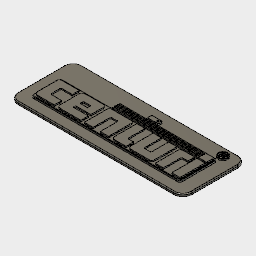
Centuri (Autodesk Fusion 360 design; units mm, degrees)
Autodesk Fusion 360 part; units mm, degrees
sketch "Sketch1" plane through (0, 0, 0) normal (0, 1, 0) x (1, 0, 0)
  spline S0 degree 3 poles (174.1224, -9.0926) (174.1224, -4.1474) (170.1072, -0.1324) (165.162, -0.1324) knots 0 0 0 0 1 1 1 1
  line L0 (165.162, -0.1324) -> (9.0926, -0.1324)
  spline S1 degree 3 poles (9.0926, -0.1324) (4.1474, -0.1324) (0.1323, -4.1474) (0.1323, -9.0926) knots 0 0 0 0 1 1 1 1
  line L1 (0.1323, -9.0926) -> (0.1323, -55.1748)
  spline S2 degree 3 poles (0.1323, -55.1748) (0.1323, -60.12) (4.1474, -64.135) (9.0926, -64.135) knots 0 0 0 0 1 1 1 1
  line L2 (9.0926, -64.135) -> (165.162, -64.135)
  spline S3 degree 3 poles (165.162, -64.135) (170.1072, -64.135) (174.1224, -60.12) (174.1224, -55.1748) knots 0 0 0 0 1 1 1 1
  line L3 (174.1224, -55.1748) -> (174.1224, -9.0926)
extrude "Extrude1" add sketch "Sketch1" along normal blind 2.5
sketch "Sketch2" plane through (0, 2.5, 0) normal (0, 1, 0) x (-1, 0, 0)
  line L0 (-174.1224, 55.1748) -> (-174.1224, 9.0926)
  spline S0 degree 3 poles (-174.1224, 9.0926) (-174.1224, 4.1474) (-170.1072, 0.1324) (-165.162, 0.1324) knots 0 0 0 0 1 1 1 1
  line L1 (-165.162, 0.1324) -> (-9.0926, 0.1324)
  spline S1 degree 3 poles (-9.0926, 0.1324) (-4.1474, 0.1324) (-0.1323, 4.1474) (-0.1323, 9.0926) knots 0 0 0 0 1 1 1 1
  line L2 (-0.1323, 9.0926) -> (-0.1323, 55.1748)
  spline S2 degree 3 poles (-0.1323, 55.1748) (-0.1323, 60.12) (-4.1474, 64.135) (-9.0926, 64.135) knots 0 0 0 0 1 1 1 1
  line L3 (-9.0926, 64.135) -> (-165.162, 64.135)
  spline S3 degree 3 poles (-165.162, 64.135) (-170.1072, 64.135) (-174.1224, 60.12) (-174.1224, 55.1748) knots 0 0 0 0 1 1 1 1
  spline S4 degree 2 poles (-15.1624, 24.5465) (-23.495, 24.5465) (-62.1665, 24.5613) knots 0 0 0 1 1 1
  spline S5 degree 2 poles (-62.1665, 24.5613) (-62.5856, 24.583) (-62.9216, 24.4382) knots 0 0 0 1 1 1
  spline S6 degree 3 poles (-62.9216, 24.4382) (-62.998, 24.4054) (-63.1803, 24.2591) (-63.2581, 24.0509) knots 0 0 0 0 1 1 1 1
  spline S7 degree 2 poles (-63.2581, 24.0509) (-63.3521, 23.7995) (-63.3351, 23.482) knots 0 0 0 1 1 1
  spline S8 degree 2 poles (-63.3351, 23.482) (-63.338, 19.0394) (-63.3351, 17.8062) knots 0 0 0 1 1 1
  spline S9 degree 3 poles (-63.3351, 17.8062) (-63.3335, 17.1487) (-63.7825, 16.1729) (-64.44, 16.1721) knots 0 0 0 0 1 1 1 1
  spline S10 degree 3 poles (-64.44, 16.1721) (-68.6437, 16.1658) (-83.8279, 16.1713) (-88.5401, 16.1711) knots 0 0 0 0 1 1 1 1
  spline S11 degree 3 poles (-88.5401, 16.1711) (-89.2008, 16.1708) (-89.5479, 16.224) (-89.5627, 15.5723) knots 0 0 0 0 1 1 1 1
  spline S12 degree 2 poles (-89.5627, 15.5723) (-89.5961, 14.1198) (-89.5627, 11.2842) knots 0 0 0 1 1 1
  spline S13 degree 3 poles (-89.5627, 11.2842) (-89.5627, 10.7958) (-89.9593, 10.3992) (-90.4478, 10.3992) knots 0 0 0 0 1 1 1 1
  line L4 (-90.4478, 10.3992) -> (-99.1457, 10.3992)
  spline S14 degree 3 poles (-99.1457, 10.3992) (-99.6341, 10.3992) (-100.0307, 10.7958) (-100.0307, 11.2842) knots 0 0 0 0 1 1 1 1
  spline S15 degree 2 poles (-100.0307, 11.2842) (-100.0021, 14.3261) (-100.0209, 15.5535) knots 0 0 0 1 1 1
  spline S16 degree 3 poles (-100.0209, 15.5535) (-100.0315, 16.242) (-100.4882, 16.1708) (-101.101, 16.1716) knots 0 0 0 0 1 1 1 1
  spline S17 degree 3 poles (-101.101, 16.1716) (-110.8882, 16.1846) (-148.8429, 16.1753) (-158.7502, 16.1721) knots 0 0 0 0 1 1 1 1
  spline S18 degree 3 poles (-158.7502, 16.1721) (-159.6421, 16.1716) (-160.4602, 17.3384) (-160.4594, 18.2301) knots 0 0 0 0 1 1 1 1
  spline S19 degree 3 poles (-160.4594, 18.2301) (-160.4576, 20.1639) (-160.4679, 26.0257) (-160.4679, 27.4458) knots 0 0 0 0 1 1 1 1
  spline S20 degree 2 poles (-160.4679, 27.4458) (-160.4674, 46.2841) (-160.4679, 50.641) knots 0 0 0 1 1 1
  spline S21 degree 3 poles (-160.4679, 50.641) (-160.4682, 53.0103) (-159.9139, 53.5406) (-157.5686, 53.5406) knots 0 0 0 0 1 1 1 1
  spline S22 degree 3 poles (-157.5686, 53.5406) (-133.3068, 53.5403) (-39.3625, 53.5421) (-15.1624, 53.5406) knots 0 0 0 0 1 1 1 1
  spline S23 degree 3 poles (-15.1624, 53.5406) (-12.6611, 53.5403) (-11.9475, 53.0579) (-11.9488, 50.641) knots 0 0 0 0 1 1 1 1
  spline S24 degree 3 poles (-11.9488, 50.641) (-11.9515, 46.2857) (-11.9491, 31.8307) (-11.9488, 27.4458) knots 0 0 0 0 1 1 1 1
  spline S25 degree 3 poles (-11.9488, 27.4458) (-11.9488, 25.0253) (-12.6291, 24.5465) (-15.1624, 24.5465) knots 0 0 0 0 1 1 1 1
extrude "Extrude2" add sketch "Sketch2" along normal blind 2 contours S4 S5 S6 S7 S8 S9 S10 S11 S12 S13 L4 S14 S15 S16 S17 S18 S19 S20 S21 S22 S23 S24 S25
sketch "Sketch3" plane through (0, 4.5, 0) normal (0, 1, 0) x (-1, 0, 0)
  spline S0 degree 3 poles (-11.9488, 27.4458) (-11.9491, 31.8307) (-11.9515, 46.2857) (-11.9488, 50.641) knots -1 -1 -1 -1 0 0 0 0
  spline S1 degree 3 poles (-11.9488, 50.641) (-11.9475, 53.0579) (-12.6611, 53.5403) (-15.1624, 53.5406) knots -1 -1 -1 -1 0 0 0 0
  spline S2 degree 3 poles (-15.1624, 53.5406) (-39.3625, 53.5421) (-133.3068, 53.5403) (-157.5686, 53.5406) knots -1 -1 -1 -1 0 0 0 0
  spline S3 degree 3 poles (-157.5686, 53.5406) (-159.9139, 53.5406) (-160.4682, 53.0103) (-160.4679, 50.641) knots -1 -1 -1 -1 0 0 0 0
  spline S4 degree 2 poles (-160.4679, 50.641) (-160.4674, 46.2841) (-160.4679, 27.4458) knots -1 -1 -1 0 0 0
  spline S5 degree 3 poles (-160.4679, 27.4458) (-160.4679, 26.0257) (-160.4576, 20.1639) (-160.4594, 18.2301) knots -1 -1 -1 -1 0 0 0 0
  spline S6 degree 3 poles (-160.4594, 18.2301) (-160.4602, 17.3384) (-159.6421, 16.1716) (-158.7502, 16.1721) knots -1 -1 -1 -1 0 0 0 0
  spline S7 degree 3 poles (-158.7502, 16.1721) (-148.8429, 16.1753) (-110.8882, 16.1846) (-101.101, 16.1716) knots -1 -1 -1 -1 0 0 0 0
  spline S8 degree 3 poles (-101.101, 16.1716) (-100.4882, 16.1708) (-100.0315, 16.242) (-100.0209, 15.5535) knots -1 -1 -1 -1 0 0 0 0
  spline S9 degree 2 poles (-100.0209, 15.5535) (-100.0021, 14.3261) (-100.0307, 11.2842) knots -1 -1 -1 0 0 0
  spline S10 degree 3 poles (-100.0307, 11.2842) (-100.0307, 10.7958) (-99.6341, 10.3992) (-99.1457, 10.3992) knots -1 -1 -1 -1 0 0 0 0
  line L0 (-99.1457, 10.3992) -> (-90.4478, 10.3992)
  spline S11 degree 3 poles (-90.4478, 10.3992) (-89.9593, 10.3992) (-89.5627, 10.7958) (-89.5627, 11.2842) knots -1 -1 -1 -1 0 0 0 0
  spline S12 degree 2 poles (-89.5627, 11.2842) (-89.5961, 14.1198) (-89.5627, 15.5723) knots -1 -1 -1 0 0 0
  spline S13 degree 3 poles (-89.5627, 15.5723) (-89.5479, 16.224) (-89.2008, 16.1708) (-88.5401, 16.1711) knots -1 -1 -1 -1 0 0 0 0
  spline S14 degree 3 poles (-88.5401, 16.1711) (-83.8279, 16.1713) (-68.6437, 16.1658) (-64.44, 16.1721) knots -1 -1 -1 -1 0 0 0 0
  spline S15 degree 3 poles (-64.44, 16.1721) (-63.7825, 16.1729) (-63.3335, 17.1487) (-63.3351, 17.8062) knots -1 -1 -1 -1 0 0 0 0
  spline S16 degree 2 poles (-63.3351, 17.8062) (-63.338, 19.0394) (-63.3351, 23.482) knots -1 -1 -1 0 0 0
  spline S17 degree 2 poles (-63.3351, 23.482) (-63.3521, 23.7995) (-63.2581, 24.0509) knots -1 -1 -1 0 0 0
  spline S18 degree 3 poles (-63.2581, 24.0509) (-63.1803, 24.2591) (-62.998, 24.4054) (-62.9216, 24.4382) knots -1 -1 -1 -1 0 0 0 0
  spline S19 degree 2 poles (-62.9216, 24.4382) (-62.5856, 24.583) (-62.1665, 24.5613) knots -1 -1 -1 0 0 0
  spline S20 degree 2 poles (-62.1665, 24.5613) (-23.495, 24.5465) (-15.1624, 24.5465) knots -1 -1 -1 0 0 0
  spline S21 degree 3 poles (-15.1624, 24.5465) (-12.6291, 24.5465) (-11.9488, 25.0253) (-11.9488, 27.4458) knots -1 -1 -1 -1 0 0 0 0
  spline S22 degree 2 poles (-32.9928, 26.8178) (-19.083, 26.7952) (-15.8247, 26.8178) knots 0 0 0 1 1 1
  spline S23 degree 3 poles (-15.8247, 26.8178) (-14.6011, 26.8261) (-13.0709, 27.9977) (-13.0639, 29.2054) knots 0 0 0 0 1 1 1 1
  spline S24 degree 3 poles (-13.0639, 29.2054) (-13.0417, 32.9886) (-13.0526, 45.265) (-13.0639, 49.042) knots 0 0 0 0 1 1 1 1
  spline S25 degree 3 poles (-13.0639, 49.042) (-13.0677, 50.37) (-14.4791, 51.9469) (-15.8247, 51.9487) knots 0 0 0 0 1 1 1 1
  spline S26 degree 2 poles (-15.8247, 51.9487) (-19.0795, 51.9532) (-32.9674, 51.9487) knots 0 0 0 1 1 1
  line L1 (-32.9674, 51.9487) -> (-32.9928, 44.3788)
  spline S27 degree 2 poles (-32.9928, 44.3788) (-24.5516, 44.3725) (-22.6517, 44.3788) knots 0 0 0 1 1 1
  spline S28 degree 3 poles (-22.6517, 44.3788) (-22.0091, 44.3809) (-21.5788, 43.4319) (-21.5873, 42.7928) knots 0 0 0 0 1 1 1 1
  spline S29 degree 3 poles (-21.5873, 42.7928) (-21.6066, 41.3105) (-21.5967, 36.9365) (-21.5873, 35.4147) knots 0 0 0 0 1 1 1 1
  spline S30 degree 3 poles (-21.5873, 35.4147) (-21.5834, 34.8089) (-22.0316, 33.8745) (-22.6453, 33.8752) knots 0 0 0 0 1 1 1 1
  spline S31 degree 2 poles (-22.6453, 33.8752) (-24.5882, 33.8783) (-32.9928, 33.8752) knots 0 0 0 1 1 1
  line L2 (-32.9928, 33.8752) -> (-32.9928, 26.8178)
  spline S32 degree 3 poles (-56.7768, 26.8178) (-53.3593, 26.806) (-42.7162, 26.8025) (-39.2193, 26.8178) knots 0 0 0 0 1 1 1 1
  spline S33 degree 3 poles (-39.2193, 26.8178) (-37.8445, 26.8237) (-35.8622, 27.8316) (-35.8661, 29.1884) knots 0 0 0 0 1 1 1 1
  spline S34 degree 3 poles (-35.8661, 29.1884) (-35.8777, 33.0541) (-35.8672, 45.7175) (-35.8661, 49.4432) knots 0 0 0 0 1 1 1 1
  spline S35 degree 3 poles (-35.8661, 49.4432) (-35.8658, 50.8266) (-37.8171, 51.9476) (-39.2193, 51.9487) knots 0 0 0 0 1 1 1 1
  spline S36 degree 2 poles (-39.2193, 51.9487) (-43.0994, 51.9508) (-59.7334, 51.9487) knots 0 0 0 1 1 1
  line L3 (-59.7334, 51.9487) -> (-59.7334, 44.3788)
  spline S37 degree 2 poles (-59.7334, 44.3788) (-47.3321, 44.3802) (-44.8507, 44.3788) knots 0 0 0 1 1 1
  spline S38 degree 3 poles (-44.8507, 44.3788) (-44.0281, 44.3781) (-44.0281, 41.943) (-44.8507, 41.944) knots 0 0 0 0 1 1 1 1
  spline S39 degree 2 poles (-44.8507, 41.944) (-47.3567, 41.9471) (-59.7334, 41.944) knots 0 0 0 1 1 1
  spline S40 degree 2 poles (-59.7334, 41.944) (-59.732, 31.8277) (-59.7334, 29.1884) knots 0 0 0 1 1 1
  spline S41 degree 3 poles (-59.7334, 29.1884) (-59.7342, 27.9349) (-58.0465, 26.8219) (-56.7768, 26.8178) knots 0 0 0 0 1 1 1 1
  line L4 (-44.6029, 37.6033) -> (-52.1177, 37.6033)
  spline S42 degree 2 poles (-52.1177, 37.6033) (-52.1195, 35.5658) (-52.1177, 35.0104) knots 0 0 0 1 1 1
  spline S43 degree 3 poles (-52.1177, 35.0104) (-52.117, 34.6915) (-51.7641, 34.3481) (-51.4621, 34.3488) knots 0 0 0 0 1 1 1 1
  spline S44 degree 3 poles (-51.4621, 34.3488) (-50.3271, 34.3526) (-46.4378, 34.3473) (-45.2915, 34.3488) knots 0 0 0 0 1 1 1 1
  spline S45 degree 3 poles (-45.2915, 34.3488) (-44.9814, 34.3496) (-44.6039, 34.683) (-44.6029, 35.0104) knots 0 0 0 0 1 1 1 1
  spline S46 degree 2 poles (-44.6029, 35.0104) (-44.6011, 35.5814) (-44.6029, 37.6033) knots 0 0 0 1 1 1
  line L5 (-63.1696, 51.9483) -> (-71.8638, 51.9483)
  spline S47 degree 2 poles (-71.8638, 51.9483) (-71.8656, 38.5103) (-71.8638, 35.6595) knots 0 0 0 1 1 1
  spline S48 degree 3 poles (-71.8638, 35.6595) (-71.8634, 34.7649) (-71.8395, 34.1505) (-72.4016, 34.1501) knots 0 0 0 0 1 1 1 1
  spline S49 degree 3 poles (-72.4016, 34.1501) (-73.5093, 34.1491) (-77.3834, 34.1456) (-78.5466, 34.1501) knots 0 0 0 0 1 1 1 1
  spline S50 degree 3 poles (-78.5466, 34.1501) (-79.1909, 34.1526) (-79.1888, 34.8162) (-79.1895, 35.6595) knots 0 0 0 0 1 1 1 1
  spline S51 degree 2 poles (-79.1895, 35.6595) (-79.1923, 38.6438) (-79.1895, 51.9071) knots 0 0 0 1 1 1
  line L6 (-79.1895, 51.9071) -> (-87.5653, 51.9483)
  spline S52 degree 2 poles (-87.5653, 51.9483) (-87.5688, 33.4546) (-87.5653, 29.1884) knots 0 0 0 1 1 1
  spline S53 degree 3 poles (-87.5653, 29.1884) (-87.5646, 28.1107) (-86.4298, 26.8171) (-85.3377, 26.8178) knots 0 0 0 0 1 1 1 1
  spline S54 degree 3 poles (-85.3377, 26.8178) (-81.607, 26.8202) (-69.4534, 26.8101) (-65.7431, 26.8178) knots 0 0 0 0 1 1 1 1
  spline S55 degree 3 poles (-65.7431, 26.8178) (-64.5697, 26.8202) (-63.1696, 28.0306) (-63.1696, 29.1884) knots 0 0 0 0 1 1 1 1
  spline S56 degree 2 poles (-63.1696, 29.1884) (-63.1689, 33.4147) (-63.1696, 51.9483) knots 0 0 0 1 1 1
  line L7 (-90.6576, 26.8178) -> (-98.9156, 26.8178)
  spline S57 degree 2 poles (-98.9156, 26.8178) (-98.9159, 40.6126) (-98.9156, 43.5182) knots 0 0 0 1 1 1
  spline S58 degree 3 poles (-98.9156, 43.5182) (-98.9152, 43.9294) (-99.3947, 44.3788) (-99.8116, 44.3788) knots 0 0 0 0 1 1 1 1
  spline S59 degree 2 poles (-99.8116, 44.3788) (-99.8559, 44.3788) (-104.8904, 44.3788) knots 0 0 0 1 1 1
  line L8 (-104.8904, 44.3788) -> (-104.946, 51.9532)
  spline S60 degree 2 poles (-104.946, 51.9532) (-96.959, 51.9452) (-94.523, 51.9532) knots 0 0 0 1 1 1
  spline S61 degree 3 poles (-94.523, 51.9532) (-90.2713, 51.9667) (-90.6439, 48.9779) (-90.6435, 47.4106) knots 0 0 0 0 1 1 1 1
  spline S62 degree 2 poles (-90.6435, 47.4106) (-90.6425, 43.2176) (-90.6576, 26.8178) knots 0 0 0 1 1 1
  line L9 (-107.072, 26.8178) -> (-115.2878, 26.8178)
  spline S63 degree 2 poles (-115.2878, 26.8178) (-115.2881, 40.5276) (-115.2878, 43.4547) knots 0 0 0 1 1 1
  spline S64 degree 3 poles (-115.2878, 43.4547) (-115.2878, 43.8323) (-115.5693, 44.3784) (-115.9521, 44.3788) knots 0 0 0 0 1 1 1 1
  spline S65 degree 3 poles (-115.9521, 44.3788) (-117.0559, 44.3791) (-120.8583, 44.3788) (-121.979, 44.3788) knots 0 0 0 0 1 1 1 1
  spline S66 degree 3 poles (-121.979, 44.3788) (-122.3375, 44.3788) (-122.508, 43.8084) (-122.5084, 43.4547) knots 0 0 0 0 1 1 1 1
  spline S67 degree 2 poles (-122.5084, 43.4547) (-122.5105, 40.5287) (-122.5084, 26.8178) knots 0 0 0 1 1 1
  line L10 (-122.5084, 26.8178) -> (-130.83, 26.8178)
  spline S68 degree 2 poles (-130.83, 26.8178) (-130.8286, 44.9394) (-130.83, 49.1325) knots 0 0 0 1 1 1
  spline S69 degree 3 poles (-130.83, 49.1325) (-130.8303, 50.3291) (-129.8661, 51.9483) (-128.543, 51.9494) knots 0 0 0 0 1 1 1 1
  spline S70 degree 3 poles (-128.543, 51.9494) (-124.6333, 51.9528) (-112.8693, 51.9521) (-109.3164, 51.9494) knots 0 0 0 0 1 1 1 1
  spline S71 degree 3 poles (-109.3164, 51.9494) (-108.0865, 51.9487) (-107.0706, 50.2577) (-107.072, 49.1328) knots 0 0 0 0 1 1 1 1
  spline S72 degree 2 poles (-107.072, 49.1328) (-107.0765, 44.9318) (-107.072, 26.8178) knots 0 0 0 1 1 1
  line L11 (-148.6286, 26.8178) -> (-148.6286, 33.5954)
  spline S73 degree 2 poles (-148.6286, 33.5954) (-144.7896, 33.5968) (-143.7112, 33.5954) knots 0 0 0 1 1 1
  spline S74 degree 3 poles (-143.7112, 33.5954) (-142.9807, 33.5943) (-142.2763, 34.5093) (-142.2756, 35.2306) knots 0 0 0 0 1 1 1 1
  spline S75 degree 2 poles (-142.2756, 35.2306) (-142.2735, 38.3037) (-142.2756, 51.9521) knots 0 0 0 1 1 1
  line L12 (-142.2756, 51.9521) -> (-134.2615, 51.9521)
  spline S76 degree 2 poles (-134.2615, 51.9521) (-134.2622, 33.6976) (-134.2615, 29.4065) knots 0 0 0 1 1 1
  spline S77 degree 3 poles (-134.2615, 29.4065) (-134.2612, 27.9849) (-136.2557, 26.8198) (-137.6963, 26.8178) knots 0 0 0 0 1 1 1 1
  spline S78 degree 2 poles (-137.6963, 26.8178) (-140.0743, 26.8143) (-148.6286, 26.8178) knots 0 0 0 1 1 1
  line L13 (-150.7694, 26.8178) -> (-159.0611, 26.8178)
  line L14 (-159.0611, 26.8178) -> (-159.0611, 51.949)
  line L15 (-159.0611, 51.949) -> (-150.7694, 51.8679)
  line L16 (-150.7694, 51.8679) -> (-150.7694, 26.8178)
  spline S79 degree 3 poles (-98.4051, 12.6404) (-98.4051, 12.3033) (-98.1313, 12.0297) (-97.7942, 12.0297) knots 0 0 0 0 1 1 1 1
  line L17 (-97.7942, 12.0297) -> (-91.45, 12.0297)
  spline S80 degree 3 poles (-91.45, 12.0297) (-91.113, 12.0297) (-90.8394, 12.3033) (-90.8394, 12.6404) knots 0 0 0 0 1 1 1 1
  line L18 (-90.8394, 12.6404) -> (-90.8394, 15.7818)
  spline S81 degree 3 poles (-90.8394, 15.7818) (-90.8394, 16.1189) (-91.113, 16.3927) (-91.45, 16.3927) knots 0 0 0 0 1 1 1 1
  line L19 (-91.45, 16.3927) -> (-97.7942, 16.3927)
  spline S82 degree 3 poles (-97.7942, 16.3927) (-98.1313, 16.3927) (-98.4051, 16.1189) (-98.4051, 15.7818) knots 0 0 0 0 1 1 1 1
  line L20 (-98.4051, 15.7818) -> (-98.4051, 12.6404)
  spline S83 degree 2 poles (-64.6658, 17.7949) (-80.3905, 17.7962) (-159.0863, 17.7949) knots 0 0 0 1 1 1
  line L21 (-159.0863, 17.7949) -> (-159.0863, 25.3701)
  spline S84 degree 2 poles (-159.0863, 25.3701) (-80.3944, 25.3701) (-64.6658, 25.3701) knots 0 0 0 1 1 1
  spline S85 degree 3 poles (-64.6658, 25.3701) (-64.173, 25.3701) (-64.1386, 24.2219) (-64.6658, 24.2219) knots 0 0 0 0 1 1 1 1
  spline S86 degree 3 poles (-64.6658, 24.2219) (-79.0329, 24.2233) (-136.3969, 24.2233) (-150.7538, 24.2219) knots 0 0 0 0 1 1 1 1
  spline S87 degree 3 poles (-150.7538, 24.2219) (-151.4642, 24.2219) (-151.4593, 23.1496) (-150.7538, 23.153) knots 0 0 0 0 1 1 1 1
  spline S88 degree 3 poles (-150.7538, 23.153) (-136.4039, 23.2243) (-78.9781, 23.1647) (-64.6658, 23.153) knots 0 0 0 0 1 1 1 1
  spline S89 degree 3 poles (-64.6658, 23.153) (-64.1649, 23.1526) (-64.1765, 22.084) (-64.6658, 22.084) knots 0 0 0 0 1 1 1 1
  spline S90 degree 3 poles (-64.6658, 22.084) (-79.0139, 22.0837) (-136.3853, 22.0789) (-150.7538, 22.084) knots 0 0 0 0 1 1 1 1
  spline S91 degree 3 poles (-150.7538, 22.084) (-151.4976, 22.084) (-151.4603, 21.0151) (-150.7538, 21.0151) knots 0 0 0 0 1 1 1 1
  spline S92 degree 3 poles (-150.7538, 21.0151) (-136.3853, 21.0141) (-78.9971, 21.0158) (-64.6658, 21.0151) knots 0 0 0 0 1 1 1 1
  spline S93 degree 3 poles (-64.6658, 21.0151) (-64.1589, 21.0148) (-64.1916, 19.9461) (-64.6658, 19.9458) knots 0 0 0 0 1 1 1 1
  spline S94 degree 3 poles (-64.6658, 19.9458) (-79.022, 19.94) (-136.3582, 19.9468) (-150.7538, 19.9458) knots 0 0 0 0 1 1 1 1
  spline S95 degree 3 poles (-150.7538, 19.9458) (-151.4023, 19.9458) (-151.4044, 18.8769) (-150.7538, 18.8769) knots 0 0 0 0 1 1 1 1
  spline S96 degree 3 poles (-150.7538, 18.8769) (-136.4039, 18.8796) (-79.0333, 18.8727) (-64.6658, 18.8769) knots 0 0 0 0 1 1 1 1
  spline S97 degree 3 poles (-64.6658, 18.8769) (-64.1625, 18.8772) (-64.167, 17.7945) (-64.6658, 17.7949) knots 0 0 0 0 1 1 1 1
extrude "Extrude3" add sketch "Sketch3" along normal blind 1.25 contours S22 S23 S24 S25 S26 L1 S27 S28 S29 S30 S31 L2 | S32 S33 S34 S35 S36 L3 S37 S38 S39 S40 S41 | L5 S47 S48 S49 S50 S51 L6 S52 S53 S54 S55 S56 | L7 S57 S58 S59 L8 S60 S61 S62 | L9 S63 S64 S65 S66 S67 L10 S68 S69 S70 S71 S72 | L11 S73 S74 S75 L12 S76 S77 S78 | L13 L14 L15 L16 | S79 L17 S80 L18 S81 L19 S82 L20 | S83 L21 S84 S85 S86 S87 S88 S89 S90 S91 S92 S93 S94 S95 S96 S97
fillet "Fillet1" radius 0.85 8 edges at (0.1323, 2.5, 32.1337) (2.758, 2.5, 61.5094) (87.1273, 2.5, 64.135) (171.4967, 2.5, 61.5094) (174.1224, 2.5, 32.1337) (171.4967, 2.5, 2.758) (87.1273, 2.5, 0.1324) (2.758, 2.5, 2.758)
fillet "Fillet2" radius 0.5 23 edges at (89.5794, 4.5, 13.774) (89.2936, 4.5, 16.116) (76.2994, 4.5, 16.1693) (63.6404, 4.5, 16.7429) (63.3366, 4.5, 19.8418) (99.7714, 4.5, 10.6585) (94.7967, 4.5, 10.3992) (89.8221, 4.5, 10.6585) (31.0797, 4.5, 24.5502) (12.6056, 4.5, 25.0884) (11.9499, 4.5, 39.0545) (12.6171, 4.5, 52.997) (86.3424, 4.5, 53.541) (159.8978, 4.5, 52.9793) (160.4676, 4.5, 42.6637) (160.463, 4.5, 23.0306) (159.9396, 4.5, 16.8665) (129.8805, 4.5, 16.1779) (100.3351, 4.5, 16.1204) (100.014, 4.5, 13.8725) (63.3243, 4.5, 23.783) (63.0894, 4.5, 24.3103) (62.5648, 4.5, 24.5414)
sketch "Sketch4" plane through (0, 2.5, 0) normal (0, 1, 0) x (-1, 0, 0)
  spline S0 degree 3 poles (-11.9488, 27.4458) (-11.9488, 25.0253) (-12.6291, 24.5465) (-15.1624, 24.5465) knots 0 0 0 0 1 1 1 1
  spline S1 degree 2 poles (-15.1624, 24.5465) (-23.495, 24.5465) (-62.1665, 24.5613) knots 0 0 0 1 1 1
  spline S2 degree 2 poles (-62.1665, 24.5613) (-62.5856, 24.583) (-62.9216, 24.4382) knots 0 0 0 1 1 1
  spline S3 degree 3 poles (-62.9216, 24.4382) (-62.998, 24.4054) (-63.1803, 24.2591) (-63.2581, 24.0509) knots 0 0 0 0 1 1 1 1
  spline S4 degree 2 poles (-63.2581, 24.0509) (-63.3521, 23.7995) (-63.3351, 23.482) knots 0 0 0 1 1 1
  spline S5 degree 2 poles (-63.3351, 23.482) (-63.338, 19.0394) (-63.3351, 17.8062) knots 0 0 0 1 1 1
  spline S6 degree 3 poles (-63.3351, 17.8062) (-63.3335, 17.1487) (-63.7825, 16.1729) (-64.44, 16.1721) knots 0 0 0 0 1 1 1 1
  spline S7 degree 3 poles (-64.44, 16.1721) (-68.6437, 16.1658) (-83.8279, 16.1713) (-88.5401, 16.1711) knots 0 0 0 0 1 1 1 1
  spline S8 degree 3 poles (-88.5401, 16.1711) (-89.2008, 16.1708) (-89.5479, 16.224) (-89.5627, 15.5723) knots 0 0 0 0 1 1 1 1
  spline S9 degree 2 poles (-89.5627, 15.5723) (-89.5961, 14.1198) (-89.5627, 11.2842) knots 0 0 0 1 1 1
  spline S10 degree 3 poles (-89.5627, 11.2842) (-89.5627, 10.7958) (-89.9593, 10.3992) (-90.4478, 10.3992) knots 0 0 0 0 1 1 1 1
  line L0 (-90.4478, 10.3992) -> (-99.1457, 10.3992)
  spline S11 degree 3 poles (-99.1457, 10.3992) (-99.6341, 10.3992) (-100.0307, 10.7958) (-100.0307, 11.2842) knots 0 0 0 0 1 1 1 1
  spline S12 degree 2 poles (-100.0307, 11.2842) (-100.0021, 14.3261) (-100.0209, 15.5535) knots 0 0 0 1 1 1
  spline S13 degree 3 poles (-100.0209, 15.5535) (-100.0315, 16.242) (-100.4882, 16.1708) (-101.101, 16.1716) knots 0 0 0 0 1 1 1 1
  spline S14 degree 3 poles (-101.101, 16.1716) (-110.8882, 16.1846) (-148.8429, 16.1753) (-158.7502, 16.1721) knots 0 0 0 0 1 1 1 1
  spline S15 degree 3 poles (-158.7502, 16.1721) (-159.6421, 16.1716) (-160.4602, 17.3384) (-160.4594, 18.2301) knots 0 0 0 0 1 1 1 1
  spline S16 degree 3 poles (-160.4594, 18.2301) (-160.4576, 20.1639) (-160.4679, 26.0257) (-160.4679, 27.4458) knots 0 0 0 0 1 1 1 1
  spline S17 degree 2 poles (-160.4679, 27.4458) (-160.4674, 46.2841) (-160.4679, 50.641) knots 0 0 0 1 1 1
  spline S18 degree 3 poles (-160.4679, 50.641) (-160.4682, 53.0103) (-159.9139, 53.5406) (-157.5686, 53.5406) knots 0 0 0 0 1 1 1 1
  spline S19 degree 3 poles (-157.5686, 53.5406) (-133.3068, 53.5403) (-39.3625, 53.5421) (-15.1624, 53.5406) knots 0 0 0 0 1 1 1 1
  spline S20 degree 3 poles (-15.1624, 53.5406) (-12.6611, 53.5403) (-11.9475, 53.0579) (-11.9488, 50.641) knots 0 0 0 0 1 1 1 1
  spline S21 degree 3 poles (-11.9488, 50.641) (-11.9515, 46.2857) (-11.9491, 31.8307) (-11.9488, 27.4458) knots 0 0 0 0 1 1 1 1
  line L1 (-0.9823, 9.0926) -> (-0.9823, 55.1748)
  spline S22 degree 3 poles (-9.0926, 63.285) (-8.6158, 63.285) (-8.139, 63.2437) (-6.3473, 62.9262) (-5.0872, 62.3534) (-3.195, 60.8423) (-2.487, 60.0006) (-1.5719, 58.3258) (-1.2872, 57.536) (-1.0312, 56.212) (-0.9823, 55.6933) (-0.9823, 55.1748) knots -1.273963 -1.273963 -1.273963 -1.273963 -1.130924 -1.130924 -0.72809 -0.72809 -0.404494 -0.404494 -0.155575 -0.155575 0 0 0 0
  line L2 (-9.0926, 63.285) -> (-165.162, 63.285)
  spline S23 degree 3 poles (-173.2724, 55.1748) (-173.2724, 55.6514) (-173.231, 56.128) (-172.9137, 57.9197) (-172.3409, 59.1799) (-170.8296, 61.0723) (-169.988, 61.7803) (-168.3132, 62.6954) (-167.5233, 62.9801) (-166.1993, 63.236) (-165.6806, 63.285) (-165.162, 63.285) knots -1.273963 -1.273963 -1.273963 -1.273963 -1.130983 -1.130983 -0.728102 -0.728102 -0.404501 -0.404501 -0.155577 -0.155577 0 0 0 0
  line L3 (-173.2724, 55.1748) -> (-173.2724, 9.0926)
  spline S24 degree 3 poles (-165.162, 0.9824) (-165.6388, 0.9824) (-166.1157, 1.0237) (-167.9073, 1.3413) (-169.1674, 1.914) (-171.0597, 3.4251) (-171.7677, 4.2668) (-172.6827, 5.9416) (-172.9675, 6.7314) (-173.2234, 8.0554) (-173.2724, 8.5741) (-173.2724, 9.0926) knots -1.273963 -1.273963 -1.273963 -1.273963 -1.130924 -1.130924 -0.728092 -0.728092 -0.404496 -0.404496 -0.155575 -0.155575 0 0 0 0
  line L4 (-165.162, 0.9824) -> (-9.0926, 0.9824)
  spline S25 degree 3 poles (-0.9823, 9.0926) (-0.9823, 8.6161) (-1.0236, 8.1394) (-1.341, 6.3478) (-1.9137, 5.0875) (-3.425, 3.1951) (-4.2667, 2.4871) (-5.9415, 1.572) (-6.7314, 1.2873) (-8.0554, 1.0314) (-8.574, 0.9824) (-9.0926, 0.9824) knots -1.273963 -1.273963 -1.273963 -1.273963 -1.130986 -1.130986 -0.728103 -0.728103 -0.404501 -0.404501 -0.155577 -0.155577 0 0 0 0
  circle A0 centre (-159.5007, 9.1533) radius 4.7474
extrude "Extrude4" add sketch "Sketch4" along normal blind 1.25 contours A0
sketch "Sketch5" plane through (0, 3.75, 0) normal (0, 1, 0) x (-1, 0, 0)
  circle A0 centre (-159.5007, 9.1533) radius 4.7474
  circle A1 centre (-159.5007, 9.1533) radius 3.625
  dimension "d11" = 7.25
  measures "d11" diameter of A1
sketch "Sketch6" plane through (0, 3.75, 0) normal (0, 1, 0) x (-1, 0, 0)
  circle A0 centre (-159.5007, 9.1533) radius 4.7474
  circle A1 centre (-159.5007, 9.1533) radius 4
  dimension "d14" = 8
  measures "d14" diameter of A1
extrude "Extrude6" cut sketch "Sketch6" against normal blind 1.25 contours A1
sketch "Sketch10" plane through (0, 2.5, 0) normal (0, 1, 0) x (-1, 0, 0)
  circle A0 centre (-159.5007, 9.1533) radius 4.7474
  spline S0 degree 3 poles (-11.9488, 27.4458) (-11.9488, 25.0253) (-12.6291, 24.5465) (-15.1624, 24.5465) knots 0 0 0 0 1 1 1 1
  spline S1 degree 2 poles (-15.1624, 24.5465) (-23.495, 24.5465) (-62.1665, 24.5613) knots 0 0 0 1 1 1
  spline S2 degree 2 poles (-62.1665, 24.5613) (-62.5856, 24.583) (-62.9216, 24.4382) knots 0 0 0 1 1 1
  spline S3 degree 3 poles (-62.9216, 24.4382) (-62.998, 24.4054) (-63.1803, 24.2591) (-63.2581, 24.0509) knots 0 0 0 0 1 1 1 1
  spline S4 degree 2 poles (-63.2581, 24.0509) (-63.3521, 23.7995) (-63.3351, 23.482) knots 0 0 0 1 1 1
  spline S5 degree 2 poles (-63.3351, 23.482) (-63.338, 19.0394) (-63.3351, 17.8062) knots 0 0 0 1 1 1
  spline S6 degree 3 poles (-63.3351, 17.8062) (-63.3335, 17.1487) (-63.7825, 16.1729) (-64.44, 16.1721) knots 0 0 0 0 1 1 1 1
  spline S7 degree 3 poles (-64.44, 16.1721) (-68.6437, 16.1658) (-83.8279, 16.1713) (-88.5401, 16.1711) knots 0 0 0 0 1 1 1 1
  spline S8 degree 3 poles (-88.5401, 16.1711) (-89.2008, 16.1708) (-89.5479, 16.224) (-89.5627, 15.5723) knots 0 0 0 0 1 1 1 1
  spline S9 degree 2 poles (-89.5627, 15.5723) (-89.5961, 14.1198) (-89.5627, 11.2842) knots 0 0 0 1 1 1
  spline S10 degree 3 poles (-89.5627, 11.2842) (-89.5627, 10.7958) (-89.9593, 10.3992) (-90.4478, 10.3992) knots 0 0 0 0 1 1 1 1
  line L0 (-90.4478, 10.3992) -> (-99.1457, 10.3992)
  spline S11 degree 3 poles (-99.1457, 10.3992) (-99.6341, 10.3992) (-100.0307, 10.7958) (-100.0307, 11.2842) knots 0 0 0 0 1 1 1 1
  spline S12 degree 2 poles (-100.0307, 11.2842) (-100.0021, 14.3261) (-100.0209, 15.5535) knots 0 0 0 1 1 1
  spline S13 degree 3 poles (-100.0209, 15.5535) (-100.0315, 16.242) (-100.4882, 16.1708) (-101.101, 16.1716) knots 0 0 0 0 1 1 1 1
  spline S14 degree 3 poles (-101.101, 16.1716) (-110.8882, 16.1846) (-148.8429, 16.1753) (-158.7502, 16.1721) knots 0 0 0 0 1 1 1 1
  spline S15 degree 3 poles (-158.7502, 16.1721) (-159.6421, 16.1716) (-160.4602, 17.3384) (-160.4594, 18.2301) knots 0 0 0 0 1 1 1 1
  spline S16 degree 3 poles (-160.4594, 18.2301) (-160.4576, 20.1639) (-160.4679, 26.0257) (-160.4679, 27.4458) knots 0 0 0 0 1 1 1 1
  spline S17 degree 2 poles (-160.4679, 27.4458) (-160.4674, 46.2841) (-160.4679, 50.641) knots 0 0 0 1 1 1
  spline S18 degree 3 poles (-160.4679, 50.641) (-160.4682, 53.0103) (-159.9139, 53.5406) (-157.5686, 53.5406) knots 0 0 0 0 1 1 1 1
  spline S19 degree 3 poles (-157.5686, 53.5406) (-133.3068, 53.5403) (-39.3625, 53.5421) (-15.1624, 53.5406) knots 0 0 0 0 1 1 1 1
  spline S20 degree 3 poles (-15.1624, 53.5406) (-12.6611, 53.5403) (-11.9475, 53.0579) (-11.9488, 50.641) knots 0 0 0 0 1 1 1 1
  spline S21 degree 3 poles (-11.9488, 50.641) (-11.9515, 46.2857) (-11.9491, 31.8307) (-11.9488, 27.4458) knots 0 0 0 0 1 1 1 1
  line L1 (-0.9823, 9.0926) -> (-0.9823, 55.1748)
  spline S22 degree 3 poles (-9.0926, 63.285) (-8.6158, 63.285) (-8.139, 63.2437) (-6.3473, 62.9262) (-5.0872, 62.3534) (-3.195, 60.8423) (-2.487, 60.0006) (-1.5719, 58.3258) (-1.2872, 57.536) (-1.0312, 56.212) (-0.9823, 55.6933) (-0.9823, 55.1748) knots -1.273963 -1.273963 -1.273963 -1.273963 -1.130924 -1.130924 -0.72809 -0.72809 -0.404494 -0.404494 -0.155575 -0.155575 0 0 0 0
  line L2 (-9.0926, 63.285) -> (-165.162, 63.285)
  spline S23 degree 3 poles (-173.2724, 55.1748) (-173.2724, 55.6514) (-173.231, 56.128) (-172.9137, 57.9197) (-172.3409, 59.1799) (-170.8296, 61.0723) (-169.988, 61.7803) (-168.3132, 62.6954) (-167.5233, 62.9801) (-166.1993, 63.236) (-165.6806, 63.285) (-165.162, 63.285) knots -1.273963 -1.273963 -1.273963 -1.273963 -1.130983 -1.130983 -0.728102 -0.728102 -0.404501 -0.404501 -0.155577 -0.155577 0 0 0 0
  line L3 (-173.2724, 55.1748) -> (-173.2724, 9.0926)
  spline S24 degree 3 poles (-165.162, 0.9824) (-165.6388, 0.9824) (-166.1157, 1.0237) (-167.9073, 1.3413) (-169.1674, 1.914) (-171.0597, 3.4251) (-171.7677, 4.2668) (-172.6827, 5.9416) (-172.9675, 6.7314) (-173.2234, 8.0554) (-173.2724, 8.5741) (-173.2724, 9.0926) knots -1.273963 -1.273963 -1.273963 -1.273963 -1.130924 -1.130924 -0.728092 -0.728092 -0.404496 -0.404496 -0.155575 -0.155575 0 0 0 0
  line L4 (-165.162, 0.9824) -> (-9.0926, 0.9824)
  spline S25 degree 3 poles (-0.9823, 9.0926) (-0.9823, 8.6161) (-1.0236, 8.1394) (-1.341, 6.3478) (-1.9137, 5.0875) (-3.425, 3.1951) (-4.2667, 2.4871) (-5.9415, 1.572) (-6.7314, 1.2873) (-8.0554, 1.0314) (-8.574, 0.9824) (-9.0926, 0.9824) knots -1.273963 -1.273963 -1.273963 -1.273963 -1.130986 -1.130986 -0.728103 -0.728103 -0.404501 -0.404501 -0.155577 -0.155577 0 0 0 0
  line L5 (-157.9472, 11.8222) -> (-157.2705, 11.8241)
  line L6 (-157.2705, 11.8241) -> (-157.2792, 6.5593)
  line L7 (-157.2792, 6.5593) -> (-161.0179, 6.552)
  spline S26 degree 2 poles (-161.0179, 6.552) (-161.3183, 6.552) (-161.4788, 6.5509) knots 0 0 0 1 1 1
  spline S27 degree 3 poles (-161.4788, 6.5509) (-161.764, 6.549) (-162.319, 7.2818) (-162.3366, 8.0212) knots 0 0 0 0 1 1 1 1
  spline S28 degree 3 poles (-162.3366, 8.0212) (-162.3591, 8.9834) (-161.7629, 9.6698) (-161.4674, 9.6733) knots 0 0 0 0 1 1 1 1
  spline S29 degree 2 poles (-161.4674, 9.6733) (-161.2646, 9.6758) (-161.006, 9.6687) knots 0 0 0 1 1 1
  line L8 (-161.006, 9.6687) -> (-161.9004, 11.8106)
  line L9 (-161.9004, 11.8106) -> (-161.2174, 11.8106)
  line L10 (-161.2174, 11.8106) -> (-160.3415, 9.6687)
  line L11 (-160.3415, 9.6687) -> (-157.9416, 9.6644)
  line L12 (-157.9416, 9.6644) -> (-157.9472, 11.8222)
  line L13 (-157.9518, 7.1869) -> (-160.8281, 7.1728)
  spline S30 degree 2 poles (-160.8281, 7.1728) (-160.9225, 7.1709) (-160.9637, 7.172) knots 0 0 0 1 1 1
  spline S31 degree 3 poles (-160.9637, 7.172) (-161.1212, 7.1761) (-161.6233, 7.3664) (-161.6228, 8.0174) knots 0 0 0 0 1 1 1 1
  spline S32 degree 3 poles (-161.6228, 8.0174) (-161.622, 8.9253) (-161.1326, 8.9573) (-160.9637, 8.9592) knots 0 0 0 0 1 1 1 1
  spline S33 degree 2 poles (-160.9637, 8.9592) (-160.8851, 8.96) (-160.8222, 8.9584) knots 0 0 0 1 1 1
  line L14 (-160.8222, 8.9584) -> (-157.9543, 8.944)
  line L15 (-157.9543, 8.944) -> (-157.9518, 7.1869)
extrude "Extrude9" add sketch "Sketch10" along normal blind 1.25 contours L5 L6 L7 S26 S27 S28 S29 L8 L9 L10 L11 L12
